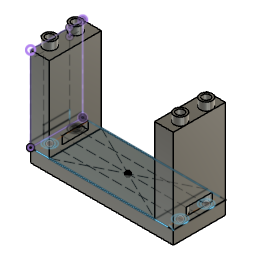
Servo Klein Halterrung (Autodesk Fusion 360 design; units mm, degrees)
Autodesk Fusion 360 part; units mm, degrees
sketch "Skizze2" plane through (0, 0, 0) normal (0, 0, 1) x (1, 0, 0)
  line L0 (0, 0) -> (54, 0)
  line L1 (54, 0) -> (54, 19.7)
  line L2 (54, 19.7) -> (0, 19.7)
  line L3 (0, 19.7) -> (0, 0)
  line L4 (51.71, 19.7) -> (2.29, 19.7)
  line L5 (2.29, 19.7) -> (2.29, 0) construction
  line L6 (2.29, 0) -> (51.71, 0)
  line L7 (51.71, 0) -> (51.71, 19.7) construction
  line L8 (51.71, 0.8354) -> (54, 0)
  line L9 (0, 19.7) -> (54, 19.7) construction
  line L10 (54, 19.7) -> (54, 9.85) construction
  line L11 (54, 9.85) -> (0, 9.85) construction
  line L12 (0, 9.85) -> (0, 19.7) construction
  line L13 (0, 14.775) -> (54, 14.775) construction
  line L14 (0, 0) -> (54, 0) construction
  line L15 (54, 0) -> (54, 4.925) construction
  line L16 (54, 4.925) -> (0, 4.925) construction
  line L17 (0, 4.925) -> (0, 0) construction
  circle A0 centre (2.29, 4.925) radius 2.29
  circle A1 centre (51.71, 14.775) radius 2.29
  circle A2 centre (51.71, 4.925) radius 2.29
  line L18 (46.95, 19.7) -> (7.05, 19.7)
  line L19 (7.05, 19.7) -> (7.05, 0)
  line L20 (7.05, 0) -> (46.95, 0)
  line L21 (46.95, 0) -> (46.95, 19.7)
  line L22 (46.95, 19.7) -> (7.05, 0) construction
  line L23 (7.05, 19.7) -> (46.95, 0) construction
  circle A3 centre (51.71, 4.925) radius 1.5
  circle A4 centre (51.71, 14.775) radius 1.5
  circle A5 centre (2.29, 4.925) radius 1.5
  circle A6 centre (2.29, 14.775) radius 1.5
  circle A7 centre (2.29, 14.775) radius 2.29
  point P0 (27, 9.85)
  dimension "d1" = 54
  dimension "d2" = 19.7
  dimension "d3" = 49.42
  dimension "d4" = 19.7
  dimension "d5" = 54
  dimension "d6" = 4.925
  dimension "d8" = 4.58
  dimension "d9" = 4.58
  dimension "d10" = 4.58
  dimension "d13" = 39.9
  dimension "d14" = 19.7
  dimension "d35" = 3
  dimension "d36" = 3
  dimension "d37" = 3
  dimension "d38" = 3
  dimension "d42" = 4.58
  constraint horizontal L0
  constraint vertical L1
  constraint horizontal L2
  constraint vertical L3
  constraint coincident L0.start L3.end
  constraint horizontal L4
  constraint perpendicular L4 L5
  constraint parallel L4 L6
  constraint parallel L5 L7
  constraint coincident L7 L8.start
  constraint horizontal L9
  constraint vertical L10
  constraint horizontal L11
  constraint vertical L12
  constraint midpoint L1 L10.end
  constraint midpoint L12 L13.start
  constraint midpoint L10 L13.end
  constraint horizontal L14
  constraint vertical L15
  constraint horizontal L16
  constraint vertical L17
  constraint coincident L5 A0.centre
  constraint coincident L16 A0.centre
  constraint coincident L13 A1.centre
  constraint coincident L7 A1.centre
  constraint coincident L16 A2.centre
  constraint coincident L7 A2.centre
  constraint horizontal L18
  constraint perpendicular L18 L19
  constraint parallel L18 L20
  constraint parallel L19 L21
  constraint coincident L22 P0
  constraint coincident L23 P0
  constraint midpoint L11 P0
  constraint concentric A2 A3
  constraint concentric A1 A4
  constraint concentric A0 A5
  constraint concentric A6 A7
  constraint coincident L13.start A7
  constraint tangent L12 A7
  measures "d1" distance of L0.start L0.end
  measures "d2" distance of L0.start L2.end
  measures "d3" distance of L5.end L6.end
  measures "d4" distance of L4.end L5.end
  measures "d5" distance of L0.start L0.end
  measures "d6" distance of L0.start L16.end
  measures "d8" diameter of A0
  measures "d9" diameter of A1
  measures "d10" diameter of A2
  measures "d13" distance of L19.end L20.end
  measures "d14" distance of L18.end L19.end
  measures "d35" diameter of A3
  measures "d36" diameter of A4
  measures "d37" diameter of A5
  measures "d38" diameter of A6
  measures "d42" diameter of A7
extrude "Extrusion1" add sketch "Skizze2" along normal blind 2.4 contours A7 | L0 L2 L3 L4 L6 L19 | L0 L2 L4 L6 L18 L19 L20 L21 | L0 L1 L2 L4 L6 L21 | A6 makes body 1
extrude "Extrusion2" add sketch "Skizze2" along normal blind 29 contours A2 | A1 | L0 L1 L2 L4 L6 L21 | A3 | A4 bodies 1
extrude "Extrusion3" add sketch "Skizze2" along normal blind 29 separate body contours A7 | A0 | L0 L2 L3 L4 L6 L19 | A5 | A6 makes body 2
extrude "Extrusion4" add sketch "Skizze2" along normal up to surface (32 mm away) contours A2 | A1 | A3 | A4 bodies 1
extrude "Extrusion5" add sketch "Skizze2" along normal up to surface (32 mm away) contours A0 | L0 L2 L3 L4 L6 L19 | A5 bodies 2 1
sketch "Skizze4" plane through (0, 0, 0) normal (1, 0, 0) x (0, 1, 0)
  line L0 (19.7, 0) -> (19.7, 32)
  line L1 (19.7, 0) -> (0, 0)
  line L2 (19.7, 0) -> (0, 0)
  line L3 (0, 0) -> (0, 32)
  line L4 (0, 32) -> (14.775, 32)
  line L5 (19.7, 32) -> (19.7, 0)
  line L6 (0, 0) -> (19.7, 0)
  line L7 (19.7, 0) -> (19.7, 2)
  line L8 (19.7, 2) -> (0, 2)
  line L9 (0, 2) -> (0, 0)
  line L10 (19.7, 0) -> (14.775, 0) construction
  line L11 (14.775, 0) -> (14.775, 29) construction
  line L12 (14.775, 29) -> (19.7, 29) construction
  line L13 (19.7, 29) -> (19.7, 0) construction
  line L14 (0, 0) -> (4.925, 0) construction
  line L15 (4.925, 0) -> (4.925, 29) construction
  line L16 (4.925, 29) -> (0, 29) construction
  line L17 (0, 29) -> (0, 0) construction
  line L18 (4.925, 2) -> (14.775, 2)
  line L19 (14.775, 2) -> (14.775, 5)
  line L20 (14.775, 5) -> (4.925, 5)
  line L21 (4.925, 5) -> (4.925, 2)
  line L22 (14.775, 32) -> (14.775, 29)
  line L23 (14.775, 29) -> (14.775, 32)
  line L24 (14.775, 32) -> (19.7, 32)
  dimension "d23" = 2
  dimension "d24" = 4.925
  dimension "d25" = 29
  dimension "d26" = 4.925
  dimension "d27" = 29
  dimension "d28" = 3
  constraint horizontal L6
  constraint vertical L7
  constraint horizontal L8
  constraint vertical L9
  constraint coincident L1.end L2.end
  constraint horizontal L10
  constraint vertical L11
  constraint horizontal L12
  constraint vertical L13
  constraint coincident L0.start L1.start
  constraint horizontal L14
  constraint vertical L15
  constraint horizontal L16
  constraint vertical L17
  constraint horizontal L18
  constraint vertical L19
  constraint horizontal L20
  constraint vertical L21
  constraint coincident L8 L18.start
  constraint coincident L15 L18.start
  measures "d23" distance of L1.end L8.end
  measures "d24" distance of L0.start L10.end
  measures "d25" distance of L0.start L12.end
  measures "d26" distance of L1.end L14.end
  measures "d27" distance of L1.end L16.end
  measures "d28" distance of L18.start L20.end
extrude "Extrusion6" cut sketch "Skizze4" along normal blind 95 contours L8 L18 L19 L20 L21 bodies 2
extrude "Extrusion7" cut sketch "Skizze2" along normal blind 25 contours L0 L2 L4 L6 L18 L19 L20 L21 bodies 2 makes body 3 at (54, 11.4917, 21)
extrude "Extrusion8" add sketch "Skizze2" against normal blind 5 contours A7 | A0 | L0 L2 L3 L4 L6 L19 | L0 L2 L4 L6 L18 L19 L20 L21 | A2 | A1 | L0 L1 L2 L4 L6 L21 | A3 | A4 | A5 | A6 bodies 2 3
extrude "Extrusion9" cut sketch "Skizze2" along normal up to surface (22 mm away) from surface at 10 contours A3 | A4 | A5 | A6 bodies 2
extrude "Extrusion10" add sketch "Skizze2" along normal blind 35 contours A7 | A0 | A2 | A1 bodies 2
extrude "Extrusion11" add 1 faces at (47.8072, 8.4333, 29) along direction (0, 0, 1) up to surface (3 mm away) on bodies 2 bodies 2
equation "d6 = ( 19.7 / 4 ) * 1 mm"
equation "d24 = ( 19.7 / 4 ) * 1 mm"
equation "d26 = ( 19.7 / 4 ) * 1 mm"
